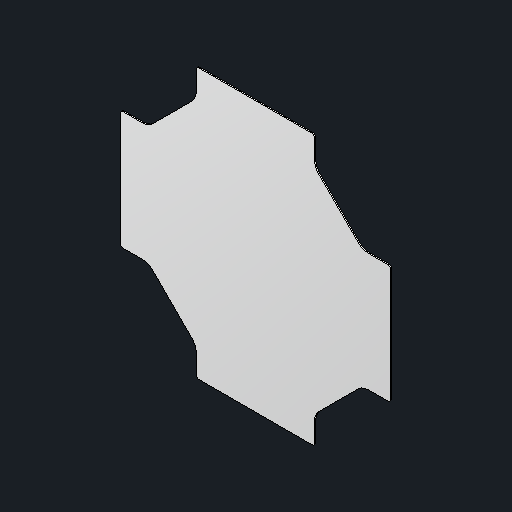
# Autodesk Inventor part: PLATE,MOUNT,ELECTRONICS
Saved by Autodesk Inventor 2026 (Build 300175000, 175)
## iProperties
Created: 2026-01-19
Part Number: PLATE,MOUNT,ELECTRONICS
Material: Aluminum 6061
Document SubType Name: Sheet Metal
Designer: Jthib
Mass: 3003.11 g
Surface Area: 7373.54 cm^2
Volume: 1112.26 cm^3
Density: 2.7 g/cm^3
Sheet Metal Rule: Default
Appearance: Aluminum - Flat
Author: Jthib
Autodesk Inventor part; units mm, degrees
ref_plane "YZ Plane" through (0, 0, 0) normal (1, 0, 0) x (0, 1, 0)
ref_plane "XZ Plane" through (0, 0, 0) normal (0, 1, 0) x (-1, 0, 0)
ref_plane "XY Plane" through (0, 0, 0) normal (0, 0, 1) x (1, 0, 0)
sketch "Sketch1" plane through (0, 0, 0) normal (0, 0, 1) x (1, 0, 0)
  line L0 (-298.45, -349.25) -> (298.45, -349.25)
  line L1 (349.25, -298.45) -> (349.25, 298.45)
  line L2 (298.45, 349.25) -> (-298.45, 349.25)
  line L3 (-349.25, 298.45) -> (-349.25, -298.45)
  line L4 (-349.25, -349.25) -> (349.25, 349.25) construction
  line L5 (349.25, -349.25) -> (-349.25, 349.25) construction
  arc A0 (349.25, 298.45) -> (298.45, 349.25) centre (298.45, 298.45) ccw
  arc A1 (-298.45, 349.25) -> (-349.25, 298.45) centre (-298.45, 298.45) ccw
  arc A2 (-349.25, -298.45) -> (-298.45, -349.25) centre (-298.45, -298.45) ccw
  arc A3 (298.45, -349.25) -> (349.25, -298.45) centre (298.45, -298.45) ccw
  point P0 (0, 0)
  dimension "d0" = 698.5
  dimension "d4" = 50.8
  measures "d0" distance of L4.end L5.end
  measures "d4" radius of A0
extrude "Plate1" add sketch "Sketch1" along normal blind 3.048
sketch "Sketch2" plane through (0, 0, 0) normal (0, 0, -1) x (-1, 0, 0)
  line L0 (-188.9125, -349.25) -> (-336.55, -349.25)
  arc A0 (-349.25, -336.55) -> (-336.55, -349.25) centre (-336.55, -336.55) ccw
  line L1 (-349.25, -336.55) -> (-349.25, -188.9125)
  line L2 (-153.035, -349.25) -> (-188.9125, -349.25)
  line L3 (-349.25, -188.9125) -> (-349.25, -153.035)
  line L4 (298.45, -349.25) -> (-298.45, -349.25) construction
  arc A1 (-270.7334, -168.4984) -> (-323.85, -190.5) centre (-292.735, -190.5) ccw construction
  line L5 (-270.7334, -168.4984) -> (-168.4984, -270.7334) construction
  arc A2 (-190.5, -323.85) -> (-168.4984, -270.7334) centre (-190.5, -292.735) ccw construction
  arc A3 (-266.2432, -164.0082) -> (-292.735, -153.035) centre (-292.735, -190.5) ccw
  line L6 (-266.2432, -164.0082) -> (-164.0082, -266.2432)
  arc A4 (-153.035, -292.735) -> (-164.0082, -266.2432) centre (-190.5, -292.735) ccw
  line L7 (-153.035, -349.25) -> (-153.035, -292.735)
  line L8 (-349.25, -153.035) -> (-292.735, -153.035)
  point P0 (0, 0)
  dimension "d10" = 6.35
  constraints: 16 end point, 10 point on circle, 5 centre point, 4 tangent, 2 perpendicular, 2 vertical, 1 collinear, 1 horizontal, 1 point on line, 15 other
  measures "d10" distance between parallel lines of L5 L6
extrude "Cut1" cut sketch "Sketch2" against normal blind 3.048
pattern_circular "Circular Pattern1" count 4 over 360 about axis through (0, 0, -10) along (0, 0, 1) of "Cut1"
fillet "Corner Round1" radius 6.35 8 edges at (-153.035, 349.25, 1.524) (349.25, -153.035, 1.524) (153.035, -349.25, 1.524) (-349.25, -153.035, 1.524) (-349.25, 153.035, 1.524) (-153.035, -349.25, 1.524) (153.035, 349.25, 1.524) (349.25, 153.035, 1.524)
equation "\"d2\" = Thickness"
equation "\"d1\" = Thickness"
equation "\"BendRadius\" = Thickness"
equation "\"BendReliefWidth\" = Thickness"
equation "\"BendReliefDepth\" = 0.5 * Thickness"
equation "\"CornerReliefSize\" = 4 * Thickness"
equation "\"MinimumRemnant\" = 2 * Thickness"
equation "\"TransitionRadius\" = BendRadius"
equation "\"JacobiRadiusSize\" = BendRadius"
equation "\"GapSize\" = Thickness"
equation "\"Thickness\" = 3.048"
body "Solid1"
